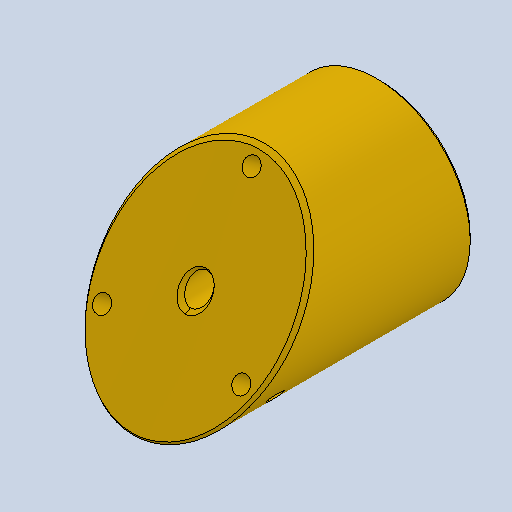
# Autodesk Inventor part: pld-sample-holder
Saved by Autodesk Inventor 2026 (Build 300175050, 175E)
## iProperties
Created: 2025-11-13
Part Number: pld-sample-holder
Material: Generic
Document SubType Name: Modeling
Designer: kuzmin
Density: 1 g/cm^3
Appearance: Gold
Author: kuzmin
Autodesk Inventor part; units mm, degrees
ref_plane "YZ Plane" through (0, 0, 0) normal (1, 0, 0) x (0, 1, 0)
ref_plane "XZ Plane" through (0, 0, 0) normal (0, 1, 0) x (-1, 0, 0)
ref_plane "XY Plane" through (0, 0, 0) normal (0, 0, 1) x (1, 0, 0)
sketch "Sketch1" plane through (0, 0, 0) normal (0, 0, 1) x (1, 0, 0)
  circle A0 centre (0, 0) radius 11.25
  dimension "d0" = 22.5
  constraints: 1 centre point, 1 coincident
  measures "d0" diameter of A0
extrude "Extrusion1" add sketch "Sketch1" along normal blind 30
sketch "Sketch3" plane through (0, 0, 0) normal (1, 0, 0) x (0, 1, 0)
  line L0 (11.25, 30) -> (-11.25, 30) projected
  line L1 (-11.25, 30) -> (11.25, 14.2453)
  line L2 (11.25, 14.2453) -> (-11.25, 30)
  line L3 (11.25, 0) -> (-11.25, 0) projected
  line L4 (11.25, 30) -> (11.25, 14.2453)
  line L5 (11.25, 0) -> (11.25, 30) projected
  point P0 (0, 0)
  dimension "d4" = 35
  constraints: 6 end point, 2 collinear, 1 vertical alignment
  measures "d4" angle of L0 L1
extrude "Extrusion2" cut sketch "Sketch3" along normal through all both and the other way through all
sketch "Sketch4" plane through (0, 0, 22.1227) normal (0, 0.5735764, 0.819152) x (1, 0, 0)
  ellipse E0 centre (0, 0) end of major axis (0, 13.7337) minor radius 11.25 projected
  spline S0 degree 5 poles (0, 15.7337) (-1.7446, 15.7336) (-3.4917, 15.3947) (-5.1439, 14.7141) (-8.2186, 12.7561) (-10.5062, 9.9092) (-11.4464, 8.2819) (-12.8901, 4.755) (-13.3732, 0.972) (-13.3731, -0.972) (-12.8903, -4.755) (-11.4463, -8.2818) (-10.5065, -9.9092) (-8.2181, -12.756) (-5.1445, -14.7141) (-3.4906, -15.3946) (0, -16.0728) (3.4906, -15.3946) (5.1445, -14.7141) (8.2181, -12.756) (10.5065, -9.9092) (11.4463, -8.2818) (12.8903, -4.755) (13.3731, -0.972) (13.3732, 0.972) (12.8901, 4.755) (11.4464, 8.2819) (10.5062, 9.9092) (8.2186, 12.7561) (5.1439, 14.7141) (3.4917, 15.3947) (1.7446, 15.7336) (0, 15.7337) knots 0 0 0 0 0 0 0.095619 0.095619 0.095619 0.197267 0.197267 0.197267 0.302733 0.302733 0.302733 0.40438 0.40438 0.40438 0.5 0.5 0.5 0.59562 0.59562 0.59562 0.697267 0.697267 0.697267 0.802733 0.802733 0.802733 0.904381 0.904381 0.904381 1 1 1 1 1 1 construction
  point P0 (0, 12.689)
  point P1 (0, 11.7337)
  point P2 (8.3618, -5)
  point P3 (-8.3618, -5)
  dimension "d7" = 2
  dimension "d15" = 5
  constraints: 1 horizontal alignment, 5 other
  measures "d15" vertical distance of point (0, 0) point (-8.362, -5)
hole "Hole1" at (0, 9.6117, 15.3925) at (8.3618, -4.0958, 24.9905) at (-8.3618, -4.0958, 24.9905) direction (0, -0.5735764, -0.819152) diameter 2 depth 5 tip angle 118
sketch "Sketch6" plane through (0, 0, 0) normal (0, 0, -1) x (-1, 0, 0)
  point P0 (0, 0)
  point P1 (0, 0)
  constraints: 1 coincident
hole "Hole2" at (0, 0, 0) direction (0, 0, 1) diameter 2.9 end through all
chamfer "Chamfer1" distance 0.4 angle 45 6 edges at (7.955, -7.955, 27.6928) (-11.25, 0, 22.1227) (7.955, 7.955, 16.5525) (-11.25, 0, 0) (0, -1.45, 0) (0, -1.45, 23.138)
body "Solid1"
